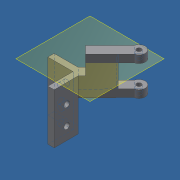
# Autodesk Inventor part: PulleyHolderXY
Saved by Autodesk Inventor 2021 (Build 250183000, 183)
## iProperties
Created: 2022-09-02
Part Number: PulleyHolderXY
Material: Generic
Document SubType Name: Modeling
Designer: Nathann
Density: 1 g/cm^3
Appearance: Default
Author: Nathann
Autodesk Inventor part; units mm, degrees
ref_plane "YZ Plane" through (0, 0, 0) normal (1, 0, 0) x (0, 1, 0)
ref_plane "XZ Plane" through (0, 0, 0) normal (0, 1, 0) x (-1, 0, 0)
ref_plane "XY Plane" through (0, 0, 0) normal (0, 0, 1) x (1, 0, 0)
sketch "Sketch1" plane through (0, 0, 0) normal (0, 0, 1) x (1, 0, 0)
  line L0 (-6.0944, 0.2158) -> (-25.1502, 0.2158)
  line L1 (-25.1502, 0.2158) -> (-25.1502, -4.7842)
  line L2 (-25.1502, -4.7842) -> (-5.1501, -4.7842)
  line L3 (-5.1501, -4.7842) -> (-5.0826, -24.7842)
  line L4 (-5.0826, -24.7842) -> (-0.0826, -24.7842)
  line L5 (-0.0826, -24.7842) -> (-0.1467, -5.8041)
  line L6 (-6.0944, 0.2158) -> (16.1426, 22.6034)
  line L7 (22.0903, 16.5836) -> (-0.1467, -5.8041)
  circle A0 centre (21.0114, 21.4658) radius 1.85
  arc A1 (22.0903, 16.5836) -> (16.1426, 22.6034) centre (21.0114, 21.4658) ccw
  dimension "d0" = 20
  dimension "d1" = 20
  dimension "d2" = 5
  dimension "d3" = 5
  dimension "d7" = 26.25
  dimension "d8" = 26.25
  dimension "d9" = 3.7
  dimension "d18" = 5
  dimension "d19" = 135
  constraints: 16 end point, 4 parallel, 2 centre point, 2 point on circle, 1 coincident, 1 horizontal, 1 perpendicular
  measures "d0" distance from line of L1.end L3
  measures "d1" distance between parallel lines of L4 L2
  measures "d2" distance of L0.end L1.end
  measures "d3" distance of L3.end L4.end
  measures "d7" distance from line of A0.centre L2
  measures "d8" distance from line of L3 A0.centre
  measures "d9" diameter of A0
  measures "d18" radius of A1
  measures "d19" angle of L7 L5
extrude "Extrusion1" add sketch "Sketch1" along normal blind 30
ref_plane "Work Plane1" through (0, 0, 24) normal (0, 0, 1) x (1, 0, 0)
sketch "Sketch3" plane through (0, 0, 24) normal (0, 0, 1) x (1, 0, 0)
  circle A0 centre (21.0114, 21.4658) radius 1.85 projected
  circle A1 centre (21.0114, 21.4658) radius 12.5
  point P0 (0, 0)
  dimension "d13" = 25
  constraints: 1 centre point, 1 coincident
  measures "d13" diameter of A1
extrude "Extrusion3" cut sketch "Sketch3" against normal blind 18
sketch "Sketch5" plane through (0, 0, 0) normal (0, 0, -1) x (-1, 0, 0)
  circle A0 centre (-21.0114, 21.4658) radius 1.85 projected
  line L0 (25.1502, -4.7842) -> (25.1502, 0.2158) projected
  line L1 (25.1502, 0.2158) -> (6.0944, 0.2158) projected
  line L2 (6.0944, 0.2158) -> (-16.1426, 22.6034) projected
  arc A1 (-16.1426, 22.6034) -> (-22.0903, 16.5836) centre (-21.0114, 21.4658) ccw projected
  line L3 (-22.0903, 16.5836) -> (0.1467, -5.8041) projected
  line L4 (0.1467, -5.8041) -> (0.0826, -24.7842) projected
  line L5 (0.0826, -24.7842) -> (5.0826, -24.7842) projected
  line L6 (5.0826, -24.7842) -> (5.1501, -4.7842) projected
  line L7 (5.1501, -4.7842) -> (25.1502, -4.7842) projected
  line L8 (0.1467, -5.8041) -> (6.0944, 0.2158)
  point P0 (0, 0)
  constraints: 2 end point
extrude "Extrusion5" add sketch "Sketch5" along normal blind 25 contours L7 L6 L5 L4 L8 L1 L0
sketch "Sketch8" plane through (-5.0826, -24.7842, -25) normal (-1, -0.0034, 0) x (0, 0, 1)
  circle A0 centre (10, 10) radius 2.25
  line L0 (55, 0) -> (0, 0) projected
  line L1 (0, 0) -> (0, 20.0001) projected
  circle A1 centre (25, 10) radius 2.25
  point P0 (25, 24.7669)
  dimension "d40" = 4.5
  dimension "d41" = 10
  dimension "d42" = 10
  dimension "d43" = 4.5
  dimension "d44" = 10
  dimension "d45" = 15
  constraints: 2 centre point
  measures "d40" diameter of A0
  measures "d41" distance from line of L0 A0.centre
  measures "d42" distance from line of L1 A0.centre
  measures "d43" diameter of A1
  measures "d44" distance from line of L0 A1.centre
  measures "d45" distance of A0.centre A1.centre
sketch "Sketch9" plane through (-25.1502, 0.2158, 30) normal (0, 1, 0) x (1, 0, 0)
  circle A0 centre (10, 45) radius 2.25
  circle A1 centre (10, 30) radius 2.25
  line L0 (0, 55) -> (19.0558, 55) projected
  line L1 (0, 0) -> (0, 55) projected
  point P0 (25.1502, 30)
  dimension "d46" = 10
  dimension "d47" = 10
  dimension "d48" = 10
  dimension "d49" = 15
  dimension "d50" = 4.5
  dimension "d51" = 4.5
  constraints: 2 centre point
  measures "d46" distance from line of L0 A0.centre
  measures "d47" distance from line of L1 A0.centre
  measures "d48" distance from line of L1 A1.centre
  measures "d49" distance of A0.centre A1.centre
  measures "d50" diameter of A0
  measures "d51" diameter of A1
extrude "Extrusion8" cut sketch "Sketch9" against normal mid plane 20
extrude "Extrusion9" cut sketch "Sketch8" against normal blind 20
sketch "Sketch10" plane through (0, 0, 30) normal (0, 0, 1) x (1, 0, 0)
  line L0 (-3.9108, 3.9108) -> (4.5333, -4.5333)
  line L1 (4.5333, -4.5333) -> (4.5333, -31.01)
  line L2 (4.5333, -31.01) -> (-28.169, -31.01)
  line L3 (-28.169, -31.01) -> (-28.169, 3.9108)
  line L4 (-28.169, 3.9108) -> (-3.9108, 3.9108)
  point P0 (0, 0)
  dimension "d56" = 135
  dimension "d57" = 0
  constraints: 10 end point, 3 perpendicular, 1 vertical
  measures "d56" angle of L0 L4
  measures "d57" distance from line of point (0, 0) L0
extrude "Extrusion10" cut sketch "Sketch10" against normal blind 15
equation "\"d43\" = d40"
equation "\"d44\" = d41"
equation "\"RodDiameter\" = 8"
equation "\"VerticalBearingOD\" = 16"
equation "\"PrintingClearance\" = 0.2"
equation "\"TubeID\" = 18"
body "Solid1"
